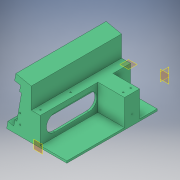
# Autodesk Inventor part: CPURightThree
Saved by Autodesk Inventor 2019 (Build 230136000, 136)
## iProperties
Created: 2019-01-04
Part Number: CPURightThree
Material: Generic
Document SubType Name: Modeling
Designer: james
Density: 1 g/cm^3
Appearance: Default(2)
Author: james
Autodesk Inventor part; units mm, degrees
ref_plane "YZ Plane" through (0, 0, 0) normal (1, 0, 0) x (0, 1, 0)
ref_plane "XZ Plane" through (0, 0, 0) normal (0, 1, 0) x (-1, 0, 0)
ref_plane "XY Plane" through (0, 0, 0) normal (0, 0, 1) x (1, 0, 0)
sketch "Sketch1" plane through (0, 0, 0) normal (0, 1, 0) x (-1, 0, 0)
  line L0 (45.712281, 188.762918) -> (-21.597719, 188.762918)
  line L1 (-21.597719, 188.762918) -> (-21.597719, -39.837082)
  line L2 (-21.597719, -39.837082) -> (45.712281, -39.837082)
  line L3 (45.712281, -39.837082) -> (45.712281, 188.762918)
  point P0 (0, 0)
  dimension "d0" = 228.6
  dimension "d1" = 67.31
  constraints: 8 end point, 2 parallel, 1 horizontal, 1 perpendicular
  measures "d0" distance of L0.end L1.end
  measures "d1" distance of L1.end L2.end
extrude "Extrusion1" add sketch "Sketch1" along normal blind 5.08
sketch "Sketch53" plane through (21.597719, 0, 188.762918) normal (0, 0, 1) x (1, 0, 0)
  line L0 (-67.31, 71.12) -> (-67.31, 5.08) projected
  line L1 (-72.39, 71.12) -> (-67.31, 71.12) projected
  line L2 (-67.31, 71.12) -> (-95.25, 71.12)
  line L3 (-95.25, 71.12) -> (-95.25, 66.04)
  line L4 (-95.25, 66.04) -> (-67.31, 66.04)
  line L5 (-67.31, 66.04) -> (-67.31, 71.12)
  line L6 (-98.425, 66.04) -> (-111.125, 66.04) projected
  line L7 (-111.125, 66.04) -> (-111.125, 71.12) projected
  point P0 (-21.597719, 0)
  point P1 (-125.73, 66.04)
  dimension "d180" = 0
  dimension "d255" = 27.94
  constraints: 8 end point, 2 parallel, 1 horizontal, 1 perpendicular
  measures "d180" distance between parallel lines of L4 L6
  measures "d255" distance of L0.start L2.end
extrude "Extrusion39" add sketch "Sketch53" against normal blind 228.6
ref_plane "Work Plane6" through (-45.712281, 71.12, -34.757082) normal (0, 1, 0) x (1, 0, 0)
sketch "Sketch60" plane through (21.597719, 0, 188.762918) normal (0, 0, 1) x (1, 0, 0)
  line L0 (-67.31, 0) -> (0, 0)
  line L1 (-147.32, 0) -> (-152.4, 0)
  line L2 (-147.32, 0) -> (-117.36365, 169.890901)
  line L3 (-98.425, 5.08) -> (-98.425, 71.12)
  line L4 (-152.4, 0) -> (-122.44365, 169.890901)
  line L5 (-117.36365, 169.890901) -> (-122.44365, 169.890901)
  point P0 (-21.597719, 0)
  point P1 (-72.39, 0)
  point P2 (-98.425, 66.04)
  dimension "d223" = 5.08
  dimension "d224" = 0
  dimension "d225" = 152.4
  dimension "d226" = 10
  dimension "d227" = 10
  constraints: 8 end point, 2 horizontal
  measures "d223" distance of L1.start L1.end
  measures "d224" distance between parallel lines of L0 L1
  measures "d225" distance of L0.end L1.end
  measures "d226" angle of L2 L3
  measures "d227" angle of L3 L4
extrude "Extrusion42" add sketch "Sketch60" against normal blind 228.6
ref_plane "Work Plane8" through (-50.792281, 0, 188.762918) normal (0, 0, 1) x (1, 0, 0)
sketch "Sketch66" plane through (-50.792281, 0, 188.762918) normal (0, 0, 1) x (1, 0, 0)
  line L0 (5.08, 71.12) -> (-22.86, 71.12)
  line L1 (-22.86, 66.04) -> (0, 66.04)
  line L2 (-17.78, 66.04) -> (-22.86, 66.04)
  line L3 (-22.86, 66.04) -> (-22.86, 162.178336)
  line L4 (-22.86, 162.178336) -> (-17.78, 162.178336)
  line L5 (-17.78, 162.178336) -> (-17.78, 66.04)
  line L6 (5.08, 71.12) -> (5.08, 5.08)
  point P0 (50.792281, 0)
  point P1 (-62.389625, 71.12)
  point P2 (-63.285366, 66.04)
  dimension "d245" = 5.08
  dimension "d252" = 22.86
  constraints: 8 end point, 2 parallel, 1 horizontal, 1 perpendicular, 1 point on line
  measures "d245" distance between parallel lines of L3 L5
  measures "d252" distance between parallel lines of L5 L6
extrude "Extrusion48" add sketch "Sketch66" against normal blind 228.6
ref_plane "Work Plane4" through (21.597719, 71.12, -58.887082) normal (1, 0, 0) x (0, 0, -1)
ref_plane "Work Plane5" through (21.597719, 66.04, -58.887082) normal (0, 0, 1) x (1, 0, 0)
ref_plane "Work Plane9" through (-50.792281, 0, 188.762918) normal (0, 0, 1) x (1, 0, 0)
sketch "Sketch76" plane through (-50.792281, 0, 188.762918) normal (0, 0, 1) x (1, 0, 0)
  line L0 (72.39, 105.3084) -> (-17.78, 124.113048)
  line L1 (-22.86, 125.172465) -> (-51.794718, 131.206702)
  line L2 (-56.69454, 132.228543) -> (-81.308126, 137.361623)
  line L3 (-81.308126, 137.361623) -> (72.39, 105.3084)
  line L4 (72.39, 105.3084) -> (72.39, 181.982006)
  line L5 (72.39, 181.982006) -> (-81.308126, 181.982006)
  line L6 (-81.308126, 137.361623) -> (-81.308126, 181.982006)
  point P0 (50.792281, 0)
  constraints: 8 end point, 2 vertical, 1 perpendicular
extrude "Extrusion56" cut sketch "Sketch76" against normal blind 312.7375
sketch "Sketch89" plane through (21.597719, 0, 188.762918) normal (0, 0, 1) x (1, 0, 0)
  line L0 (-67.31, 71.12) -> (-90.17, 71.12) projected
  line L1 (-67.31, 66.04) -> (-67.31, 71.12) projected
  line L2 (-67.31, 71.12) -> (-72.39, 71.12)
  line L3 (-72.39, 71.12) -> (-72.39, 0)
  line L4 (-72.39, 0) -> (-67.31, 0)
  line L5 (-67.31, 0) -> (-67.31, 71.12)
  point P0 (-21.597719, 0)
  dimension "d326" = 5.08
  constraints: 8 end point, 2 parallel, 1 horizontal, 1 perpendicular
  measures "d326" distance between parallel lines of L5 L3
extrude "Extrusion65" add sketch "Sketch89" against normal blind 228.6
sketch "Sketch90" plane through (21.597719, 0, 188.762918) normal (0, 0, 1) x (1, 0, 0)
  line L0 (-152.4, 0) -> (-129.08454, 132.228543)
  line L1 (-124.184718, 131.206702) -> (-129.08454, 132.228543)
  line L2 (-124.184718, 131.206702) -> (-147.32, 0)
  line L3 (-90.17, 124.113048) -> (-95.25, 125.172465)
  line L4 (-90.17, 124.113048) -> (-90.17, 71.12)
  line L5 (-129.08454, 132.228543) -> (-90.17, 124.113048)
  line L6 (-90.17, 124.113048) -> (-90.17, 118.923755)
  line L7 (-90.17, 118.923755) -> (-129.967099, 127.223305)
  line L8 (-129.08454, 132.228543) -> (-129.967099, 127.223305)
  point P0 (-21.597719, 0)
  dimension "d329" = 5.08
  constraints: 8 end point, 2 point on line, 1 parallel
  measures "d329" distance between parallel lines of L5 L7
extrude "Extrusion66" add sketch "Sketch90" against normal blind 228.6
sketch "Sketch91" plane through (-45.712281, 5.08, 188.762918) normal (0, 0, 1) x (1, 0, 0)
  line L0 (0, 0) -> (0, 66.04)
  line L1 (-5.08, -5.08) -> (67.31, -5.08)
  line L2 (-85.09, -5.08) -> (-61.77454, 127.148543)
  line L3 (-80.01, -5.08) -> (-85.09, -5.08)
  line L4 (0, 66.04) -> (-22.86, 66.04)
  line L5 (-22.86, 119.033048) -> (-22.86, 66.04)
  line L6 (-22.86, 119.033048) -> (-61.77454, 127.148543)
  line L7 (0, 66.04) -> (0, 0)
  line L8 (0, 66.04) -> (0, -5.08)
  line L9 (67.31, -5.08) -> (-5.08, -5.08)
  line L10 (-85.09, -5.08) -> (0, -5.08)
  line L11 (-80.01, -5.08) -> (-85.09, -5.08)
  line L12 (-61.77454, 127.148543) -> (-22.86, 119.033048)
  line L13 (-85.09, -5.08) -> (-61.77454, 127.148543)
  line L14 (-61.77454, 127.148543) -> (-22.86, 119.033048)
  line L15 (-22.86, 119.033048) -> (-22.86, 66.04)
  line L16 (-22.86, 119.033048) -> (-22.86, 66.04)
  line L17 (-22.86, 66.04) -> (0, 66.04)
  line L18 (-22.86, 66.04) -> (0, 66.04)
  point P0 (45.712281, -5.08)
  constraints: 12 end point, 2 collinear, 2 perpendicular
extrude "Extrusion67" add sketch "Sketch91" against normal blind 5.08
sketch "Sketch92" plane through (21.597719, 5.08, -39.837082) normal (0, 0, -1) x (-1, 0, 0)
  line L0 (67.31, 66.04) -> (67.31, 0)
  line L1 (0, -5.08) -> (72.39, -5.08)
  line L2 (152.4, -5.08) -> (129.08454, 127.148543)
  line L3 (129.08454, 127.148543) -> (90.17, 119.033048)
  line L4 (90.17, 119.033048) -> (90.17, 66.04)
  line L5 (90.17, 66.04) -> (67.31, 66.04)
  line L6 (152.4, -5.08) -> (129.08454, 127.148543)
  line L7 (129.08454, 127.148543) -> (90.17, 119.033048)
  line L8 (90.17, 119.033048) -> (90.17, 66.04)
  line L9 (90.17, 66.04) -> (67.31, 66.04)
  line L10 (67.31, 66.04) -> (67.31, -5.08)
  line L11 (129.08454, 127.148543) -> (152.4, -5.08)
  line L12 (152.4, -5.08) -> (67.31, -5.08)
  line L13 (152.4, -5.08) -> (0, -5.08)
  point P0 (21.597719, -5.08)
  constraints: 12 end point, 3 collinear, 1 perpendicular
extrude "Extrusion68" add sketch "Sketch92" against normal blind 5.08
sketch "Sketch93" plane through (21.597719, 5.08, -39.837082) normal (0, 0, -1) x (-1, 0, 0)
  line L0 (67.31, 66.04) -> (67.31, 0) projected
  line L1 (0, -5.08) -> (152.4, -5.08) projected
  point P0 (21.597719, -5.08)
  point P1 (118.11, 20.32)
  point P2 (118.11, 45.72)
  dimension "d336" = 50.8
  dimension "d337" = 50.8
  dimension "d338" = 25.4
  dimension "d339" = 25.4
  measures "d336" distance from line of L0 point (118.11, 20.32)
  measures "d337" distance from line of L0 point (118.11, 45.72)
  measures "d338" distance from line of L1 point (118.11, 20.32)
  measures "d339" distance of point (118.11, 45.72) point (118.11, 20.32)
hole "Hole14" at (-96.512281, 25.4, -39.837082) at (-96.512281, 50.8, -39.837082) direction (0, 0, 1) diameter 3.302 end through all
sketch "Sketch94" plane through (-45.712281, 71.12, 188.762918) normal (0, 1, 0) x (1, 0, 0)
  line L0 (0, 0) -> (0, 228.6) projected
  line L1 (-22.86, 228.6) -> (-22.86, 0) projected
  line L2 (-22.86, 228.6) -> (0, 228.6) projected
  line L3 (67.31, 0) -> (67.31, 228.6) projected
  line L4 (-22.86, 228.6) -> (-22.86, 0) projected
  line L5 (-22.86, 146.05) -> (67.31, 146.05)
  line L6 (67.31, 146.05) -> (67.31, 184.15)
  line L7 (67.31, 184.15) -> (-22.86, 184.15)
  line L8 (-22.86, 184.15) -> (-22.86, 146.05)
  point P0 (45.712281, 188.762918)
  dimension "d347" = 44.45
  dimension "d348" = 38.1
  constraints: 8 end point, 2 parallel, 2 point on line, 1 horizontal, 1 perpendicular
  measures "d347" distance between parallel lines of L7 L2
  measures "d348" distance between parallel lines of L5 L7
extrude "Extrusion69" add sketch "Sketch94" against normal blind 5.08 contours L5 L1 L7 L0 | L0 L7 L3 L5
sketch "Sketch95" plane through (21.597719, 71.12, 42.712918) normal (1, 0, 0) x (0, 0, -1)
  line L0 (0, 0) -> (38.1, 0) projected
  line L1 (38.1, 0) -> (38.1, -5.08) projected
  line L2 (0, 0) -> (0, -5.08) projected
  line L3 (-146.05, -71.12) -> (82.55, -71.12) projected
  line L4 (-140.97, -71.12) -> (77.47, -71.12) projected
  line L5 (0, 0) -> (5.08, 0)
  line L6 (5.08, 0) -> (5.08, -71.12)
  line L7 (5.08, -71.12) -> (0, -71.12)
  line L8 (0, -71.12) -> (0, 0)
  line L9 (38.1, 0) -> (33.02, 0)
  line L10 (33.02, 0) -> (33.02, -71.12)
  line L11 (33.02, -71.12) -> (38.1, -71.12)
  line L12 (38.1, -71.12) -> (38.1, 0)
  point P0 (42.712918, -71.12)
  dimension "d351" = 5.08
  dimension "d352" = 5.08
  constraints: 16 end point, 4 parallel, 2 horizontal, 2 perpendicular, 2 point on line
  measures "d351" distance between parallel lines of L10 L12
  measures "d352" distance between parallel lines of L8 L6
extrude "Extrusion70" add sketch "Sketch95" against normal blind 69.5325 contours L0 L6 L3 L8 L2 | L0 L1 L12 L3 L10
sketch "Sketch96" plane through (21.597719, 0, 188.762918) normal (1, 0, 0) x (0, 0, -1)
  line L0 (179.07, 66.04) -> (179.07, 5.08) projected
  line L1 (151.13, 5.08) -> (151.13, 66.04) projected
  line L2 (0, 0) -> (228.6, 0) projected
  line L3 (5.08, 0) -> (223.52, 0) projected
  line L4 (151.13, 5.08) -> (179.07, 5.08)
  line L5 (179.07, 5.08) -> (179.07, 0)
  line L6 (179.07, 0) -> (151.13, 0)
  line L7 (151.13, 0) -> (151.13, 5.08)
  point P0 (188.762918, 0)
  constraints: 8 end point, 2 parallel, 1 horizontal, 1 perpendicular, 1 point on line
extrude "Extrusion71" cut sketch "Sketch96" against normal blind 66.3575
sketch "Sketch97" plane through (21.597719, 5.08, 4.612918) normal (1, 0, 0) x (0, 0, -1)
  line L0 (-38.1, 66.04) -> (0, 66.04) projected
  line L1 (0, 66.04) -> (0, 0) projected
  line L2 (-38.1, 66.04) -> (-38.1, 0) projected
  line L3 (-5.08, -5.08) -> (-33.02, -5.08) projected
  line L4 (-179.07, -5.08) -> (39.37, -5.08) projected
  line L5 (-38.1, 66.04) -> (0, 66.04)
  line L6 (0, 66.04) -> (0, -5.08)
  line L7 (0, -5.08) -> (-38.1, -5.08)
  line L8 (-38.1, -5.08) -> (-38.1, 66.04)
  point P0 (4.612918, -5.08)
  constraints: 8 end point, 2 parallel, 1 horizontal, 1 perpendicular, 1 point on line
extrude "Extrusion72" add sketch "Sketch97" against normal blind 5.08
sketch "Sketch101" plane through (-45.712281, 5.08, 183.682918) normal (0, 0, -1) x (-1, 0, 0)
  line L0 (5.08, 60.96) -> (27.94, 60.96)
  line L1 (5.08, 60.96) -> (5.08, -5.08)
  line L2 (5.08, -5.08) -> (5.08, 60.96)
  line L3 (5.08, -5.08) -> (5.08, 60.96)
  line L4 (5.08, 60.96) -> (5.08, 46.584263)
  line L5 (5.08, 46.584263) -> (27.94, 60.96)
  line L6 (27.870815, 61.070017) -> (5.08, 60.96)
  point P0 (-45.712281, -5.08)
  constraints: 6 end point, 1 point on line
extrude "Extrusion73" add sketch "Sketch101" along normal blind 219.3925
sketch "Sketch98" plane through (21.597719, 0, 188.762918) normal (1, 0, 0) x (0, 0, -1)
  line L0 (184.15, 71.12) -> (184.15, 5.08) projected
  line L1 (0, 0) -> (228.6, 0) projected
  point P0 (188.762918, 0)
  point P1 (165.1, 25.4)
  dimension "d359" = 19.05
  dimension "d360" = 25.4
  measures "d359" distance from line of point (165.1, 25.4) L0
  measures "d360" distance from line of L1 point (165.1, 25.4)
hole "Hole15" at (21.597719, 25.4, 23.662918) direction (-1, 0, 0) diameter 3.302 depth 25.4 tip angle 118.1875
sketch "Sketch99" plane through (-68.572281, 71.12, 188.762918) normal (0, 1, 0) x (1, 0, 0)
  line L0 (22.86, 0) -> (22.86, 146.05) projected
  line L1 (22.86, 0) -> (0, 0) projected
  point P0 (68.572281, 188.762918)
  point P1 (10.7696, 12.7)
  point P2 (10.7696, 88.9)
  dimension "d368" = 12.0904
  dimension "d369" = 12.0904
  dimension "d370" = 12.7
  dimension "d371" = 76.2
  measures "d368" distance from line of L0 point (10.77, 88.9)
  measures "d369" distance from line of L0 point (10.77, 12.7)
  measures "d370" distance from line of L1 point (10.77, 12.7)
  measures "d371" distance of point (10.77, 88.9) point (10.77, 12.7)
hole "Hole16" at (-57.802681, 71.12, 176.062918) at (-57.802681, 71.12, 99.862918) direction (0, -1, 0) diameter 3.302 depth 25.4 tip angle 118.1875
sketch "Sketch100" plane through (-68.572281, 71.12, 188.762918) normal (0, 1, 0) x (1, 0, 0)
  line L0 (22.86, 146.05) -> (90.17, 146.05) projected
  line L1 (90.17, 184.15) -> (22.86, 184.15) projected
  line L2 (90.17, 146.05) -> (90.17, 184.15) projected
  point P0 (68.572281, 188.762918)
  point P1 (77.47, 155.575)
  point P2 (77.47, 174.625)
  dimension "d379" = 9.525
  dimension "d380" = 9.525
  dimension "d381" = 12.7
  dimension "d382" = 12.7
  measures "d379" distance from line of L0 point (77.47, 155.575)
  measures "d380" distance from line of L1 point (77.47, 174.625)
  measures "d381" distance from line of L2 point (77.47, 174.625)
  measures "d382" distance from line of L2 point (77.47, 155.575)
hole "Hole17" at (8.897719, 71.12, 33.187918) at (8.897719, 71.12, 14.137918) direction (0, -1, 0) diameter 3.302 depth 25.4 tip angle 118.1875
sketch "Sketch102" plane through (-130.802281, 0, -39.837082) normal (-0.9848078, 0.1736482, 0) x (0, 0, 1)
  line L0 (0, 116.84) -> (228.6, 116.84)
  line L1 (228.6, 116.84) -> (228.6, 17.78)
  line L2 (228.6, 17.78) -> (0, 17.78)
  line L3 (0, 17.78) -> (0, 116.84)
  line L4 (228.6, 0) -> (228.6, 134.268382)
  line L5 (228.6, 0) -> (0, 0)
  point P0 (39.837082, 22.713578)
  dimension "d392" = 0
  dimension "d393" = 228.6
  dimension "d394" = 17.78
  dimension "d395" = 99.06
  constraints: 8 end point, 2 parallel, 1 horizontal, 1 perpendicular
  measures "d392" distance between parallel lines of L4 L1
  measures "d393" distance between parallel lines of L1 L3
  measures "d394" distance between parallel lines of L5 L2
  measures "d395" distance between parallel lines of L0 L2
extrude "Extrusion74" cut sketch "Sketch102" against normal blind 15.24
sketch "Sketch103" plane through (-45.712281, 5.08, 183.682918) normal (0, 0, -1) x (-1, 0, 0)
  line L0 (77.075716, 11.561151) -> (66.994065, 9.783484)
  line L1 (66.994065, 9.783484) -> (49.792477, 107.33854)
  line L2 (49.792477, 107.33854) -> (59.874128, 109.116207)
  arc A0 (77.075716, 11.561151) -> (77.075716, 11.561151) centre (74.555303, 11.116734) ccw
  line L3 (77.075716, 11.561151) -> (77.737316, 7.809033)
  line L4 (66.994065, 9.783484) -> (82.002535, 12.429882)
  line L5 (77.737316, 7.809033) -> (63.903547, 5.369767)
  line L6 (63.903547, 5.369767) -> (45.37876, 110.429058)
  line L7 (45.37876, 110.429058) -> (59.212528, 112.868324)
  line L8 (57.757277, 121.121463) -> (59.874128, 109.116207)
  line L9 (59.874128, 109.116207) -> (59.212528, 112.868324)
  line L10 (59.874128, 109.116207) -> (49.792477, 107.33854)
  line L11 (49.792477, 107.33854) -> (66.994065, 9.783484)
  line L12 (49.792477, 107.33854) -> (66.994065, 9.783484)
  line L13 (66.994065, 9.783484) -> (77.075716, 11.561151)
  point P0 (-45.712281, -5.08)
  dimension "d398" = 3.81
  dimension "d399" = 3.81
  dimension "d400" = 3.81
  constraints: 16 end point, 4 perpendicular, 4 point on line, 3 collinear, 2 point on circle, 1 centre point
  measures "d398" distance between parallel lines of L5 L0
  measures "d399" distance between parallel lines of L6 L1
  measures "d400" distance between parallel lines of L2 L7
extrude "Extrusion75" add sketch "Sketch103" along normal blind 164.465 contours A0 L0 | L3 L5 L6 L7 L8 L2 L1 L0 A0 picked at (74.022986, 10.082997)
sketch "Sketch105" plane through (-45.712281, 5.08, 188.762918) normal (1, 0, 0) x (0, 0, -1)
  line L0 (36.474148, 32.389253) -> (122.561017, 33.507264) construction
  line L1 (36.746073, 11.451052) -> (122.832941, 12.569063)
  line L2 (122.289092, 54.445465) -> (36.202223, 53.327454)
  arc A0 (36.202223, 53.327454) -> (36.746073, 11.451052) centre (36.474148, 32.389253) ccw
  arc A1 (122.832941, 12.569063) -> (122.289092, 54.445465) centre (122.561017, 33.507264) ccw
  point P0 (188.762918, -5.08)
  point P1 (79.517582, 32.948258)
  constraints: 8 end point, 4 point on circle, 4 tangent, 2 centre point, 1 midpoint, 1 parallel
extrude "Extrusion77" cut sketch "Sketch105" against normal blind 5.08
sketch "Sketch106" plane through (-115.793811, -2.646398, -39.837082) normal (-0.9848078, 0.1736482, 0) x (0, 0, 1)
  line L0 (228.6, 116.84) -> (228.6, 17.78) projected
  line L1 (68.58, 33.02) -> (228.6, 33.02)
  line L2 (228.6, 33.02) -> (228.6, 101.6)
  line L3 (228.6, 101.6) -> (68.58, 101.6)
  line L4 (68.58, 101.6) -> (68.58, 33.02)
  line L5 (228.6, 17.78) -> (0, 17.78) projected
  line L6 (0, 116.84) -> (228.6, 116.84) projected
  line L7 (68.58, 17.78) -> (68.58, 116.84) projected
  point P0 (39.837082, 22.713578)
  dimension "d407" = 15.24
  dimension "d408" = 15.24
  dimension "d409" = 0
  constraints: 8 end point, 2 parallel, 1 horizontal, 1 perpendicular, 1 point on line
  measures "d407" distance between parallel lines of L1 L5
  measures "d408" distance between parallel lines of L6 L3
  measures "d409" distance between parallel lines of L7 L4
extrude "Extrusion78" cut sketch "Sketch106" against normal blind 5.08 contours L0 L1 L4 L3
sketch "Sketch107" plane through (-45.712281, 5.08, 188.762918) normal (0, 0, 1) x (1, 0, 0)
  line L0 (-64.347667, 24.791954) -> (-66.994065, 9.783484)
  line L1 (-59.344844, 23.909821) -> (-64.347667, 24.791954)
  line L2 (-52.438875, 92.330069) -> (-47.436052, 91.447937)
  line L3 (-49.792477, 107.33854) -> (-52.438875, 92.330069)
  line L4 (-66.994065, 9.783484) -> (-49.792477, 107.33854)
  line L5 (-52.438875, 92.330069) -> (-48.686757, 91.66847)
  line L6 (-49.792477, 107.33854) -> (-52.438875, 92.330069)
  line L7 (-47.436052, 91.447937) -> (-48.686757, 91.66847)
  line L8 (-52.438875, 92.330069) -> (-48.686757, 91.66847)
  line L9 (-48.686757, 91.66847) -> (-46.040359, 106.67694)
  line L10 (-48.686757, 91.66847) -> (-45.37876, 110.429058)
  line L11 (-49.792477, 107.33854) -> (-46.040359, 106.67694)
  line L12 (-64.347667, 24.791954) -> (-60.595549, 24.130354)
  line L13 (-64.347667, 24.791954) -> (-60.595549, 24.130354)
  line L14 (-64.347667, 24.791954) -> (-66.994065, 9.783484)
  line L15 (-63.903547, 5.369767) -> (-60.595549, 24.130354)
  line L16 (-63.241948, 9.121884) -> (-66.994065, 9.783484)
  line L17 (-63.241948, 9.121884) -> (-60.595549, 24.130354)
  point P0 (45.712281, -5.08)
  constraints: 16 end point, 3 collinear, 3 perpendicular, 2 point on line
extrude "Extrusion79" add sketch "Sketch107" against normal blind 228.6
equation "\"d2\" = WallWidth"
equation "\"d223\" = WallWidth"
equation "\"d245\" = WallWidth"
equation "\"d326\" = WallWidth"
equation "\"d329\" = WallWidth"
equation "\"d332\" = WallWidth"
equation "\"d334\" = WallWidth"
equation "\"d349\" = WallWidth"
equation "\"d351\" = WallWidth"
equation "\"d352\" = WallWidth"
equation "\"d357\" = WallWidth"
equation "\"DSLength\" = 1371.6"
equation "\"DSWidth\" = 304.8"
equation "\"DCDeckHeight\" = 76.2"
equation "\"WallWidth\" = 5.08"
equation "\"EdgeAngle\" = 10deg"
equation "\"LengthCuts\" = 152.4"
equation "\"WidthCuts\" = 50.8"
equation "\"PartLength\" = 228.6"
equation "\"PartWidth\" = 152.4"
equation "\"BoltHoldDiam\" = 6.35"
equation "\"ControlPlateLength\" = 228.6"
equation "\"ControlPlateWidth\" = 228.6"
equation "\"ControlPlateShelfLength\" = 19.05"
equation "\"ControlHoleLength\" = 190.5"
equation "\"ControlHoleWidth\" = 190.5"
equation "\"ControlHoleFromSide\" = 63.5"
equation "\"ControlHoleBoltHoleMid\" = 9.525"
equation "\"CPDeckHeight\" = 71.12"
equation "\"CPFromSide\" = 63.5"
equation "\"CPFromBack\" = 63.5"
equation "\"DU1CHWidth\" = 69.85"
equation "\"DU1CHLength\" = 146.05"
equation "\"ControlPlateScrewLength\" = 76.2"
equation "\"DSBackHeight\" = 127"
equation "\"BackShelf\" = 25.4"
equation "\"MainAngle\" = 168.22deg"
equation "\"CPDWidthHole\" = 120.65"
equation "\"CPDLengthHole\" = 146.05"
equation "\"DownBackHeight\" = 130.7084"
body "Solid1"
